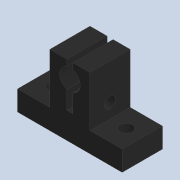
# Autodesk Inventor part: 0008-10-020 Suport Axa Y
Saved by Autodesk Inventor 2020 (Build 240168000, 168)
## iProperties
Created: 2021-02-27
Part Number: 0008-10-020 Suport Axa Y
Material: Generic
Document SubType Name: Modeling
Designer: Iulian Bors
Density: 1 g/cm^3
Appearance: Default
Description: Suport Axa
Mass: 15.8533 g
Surface Area: 63.9613 cm^2
Volume: 15.8533 cm^3
Author: Iulian Bors
Subject: 020
Autodesk Inventor part; units mm, degrees
ref_plane "YZ Plane" through (0, 0, 0) normal (1, 0, 0) x (0, 1, 0)
ref_plane "XZ Plane" through (0, 0, 0) normal (0, 1, 0) x (-1, 0, 0)
ref_plane "XY Plane" through (0, 0, 0) normal (0, 0, 1) x (1, 0, 0)
sketch "Sketch1" plane through (0, 0, 0) normal (0, 0, 1) x (1, 0, 0)
  line L0 (-28, 5) -> (28, 5)
  line L1 (28, 5) -> (28, -5)
  line L2 (28, -5) -> (-28, -5)
  line L3 (-28, -5) -> (-28, 5)
  line L4 (-10, 30) -> (10, 30)
  line L5 (10, 30) -> (10, 5)
  line L6 (10, 5) -> (-10, 5)
  line L7 (-10, 5) -> (-10, 30)
  circle A0 centre (0, 22) radius 5.15
  line L8 (-1.5, 30) -> (1.5, 30)
  line L9 (1.5, 30) -> (1.5, 8)
  line L10 (1.5, 8) -> (-1.5, 8)
  line L11 (-1.5, 8) -> (-1.5, 30)
  point P0 (0, 0)
  point P1 (-28, 0)
  point P2 (0, 5)
  point P3 (0, 30)
  point P4 (0, 30)
  point P5 (-1.5, 17.0733)
  point P6 (-1.5, 26.9267)
  point P7 (-1.5, 30)
  point P8 (-10, 5)
  point P9 (10, 5)
  point P10 (1.5, 30)
  point P11 (1.5, 26.9267)
  point P12 (1.5, 17.0733)
  dimension "d0" = 10
  dimension "d1" = 20
  dimension "d2" = 10.3
  dimension "d3" = 17
  dimension "d4" = 8
  dimension "d5" = 3
  dimension "d6" = 14
  dimension "d7" = 18
  constraints: 24 end point, 6 parallel, 4 midpoint, 3 horizontal, 3 perpendicular, 3 vertical alignment, 2 collinear, 1 centre point, 1 coincident, 1 horizontal alignment
  measures "d0" distance of L2.end L0.start
  measures "d1" distance of L4.start L4.end
  measures "d2" diameter of A0
  measures "d3" distance from line of L0 A0.centre
  measures "d4" distance from line of A0.centre L4
  measures "d5" distance between parallel lines of L11 L9
  measures "d6" distance from line of L10 A0.centre
  measures "d7" distance between parallel lines of L1 L5
extrude "Extrusion1" add sketch "Sketch1" along normal mid plane 20 contours L0 L1 L2 L3 | L7 L4 L11 A0 L10 L9 L5 L0
sketch "Sketch2" plane through (10, 5, 10) normal (0, 1, 0) x (1, 0, 0)
  line L0 (0, 20) -> (18, 20) projected
  line L1 (-38, 20) -> (-20, 20) projected
  line L2 (-38, 20) -> (-38, 0) projected
  line L3 (18, 20) -> (18, 0) projected
  point P0 (-10, 10)
  point P1 (-30, 10)
  point P2 (10, 10)
  point P3 (-38, 10)
  point P4 (18, 10)
  dimension "d25" = 8
  dimension "d26" = 8
  constraints: 2 horizontal alignment, 2 midpoint
  measures "d25" distance from line of L3 point (10, 10)
  measures "d26" distance from line of point (-30, 10) L2
hole "Hole1" at (-20, 5, 0) at (20, 5, 0) direction (0, -1, 0) diameter 6 end through all
sketch "Sketch3" plane through (10, 5, 10) normal (1, 0, 0) x (0, 0, -1)
  line L0 (20, 25) -> (0, 25) projected
  circle A0 centre (10, 7.0733) radius 2.75
  line L1 (20, 25) -> (0, 25) projected
  line L2 (0, 25) -> (8, 25)
  line L3 (8, 25) -> (8, 0)
  line L4 (8, 0) -> (0, 0)
  line L5 (0, 0) -> (0, 25)
  line L6 (20, 0) -> (0, 0) projected
  line L7 (12, 25) -> (20, 25)
  line L8 (20, 25) -> (20, 0)
  line L9 (20, 0) -> (12, 0)
  line L10 (12, 0) -> (12, 25)
  line L11 (20, 25) -> (20, 0) projected
  line L12 (20, 12.0733) -> (0, 12.0733) projected
  point P0 (10, -5)
  point P1 (10, 25)
  point P2 (12, 0)
  dimension "d18" = 5.5
  dimension "d19" = 8
  dimension "d21" = 8
  dimension "d24" = 5
  constraints: 16 end point, 4 collinear, 4 parallel, 2 horizontal, 2 perpendicular, 1 centre point, 1 coincident, 1 midpoint, 1 vertical alignment
  measures "d18" diameter of A0
  measures "d19" distance between parallel lines of L3 L5
  measures "d21" distance between parallel lines of L8 L10
  measures "d24" distance from line of point (10, 7.073) L12
extrude "Extrusion2" cut sketch "Sketch3" against normal through all contours L10 A0 L3 | A0 L10 | L3 A0
equation "\"d21\" = d19"
body "Solid1"
